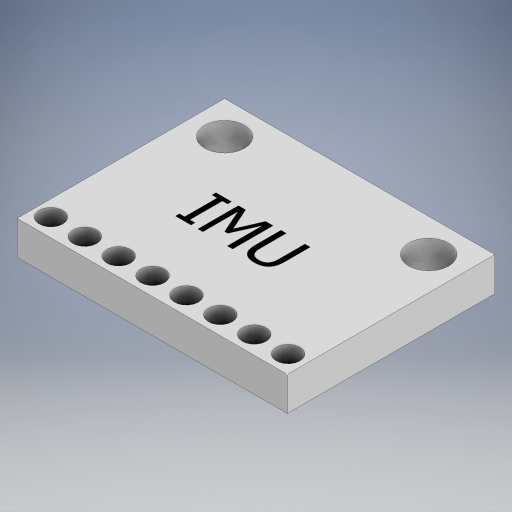
# Autodesk Inventor part: IMU_temp
Saved by Autodesk Inventor 2024 (Build 280153000, 153)
## iProperties
Created: 2025-01-15
Part Number: IMU_temp
Material: Generic
Document SubType Name: Modeling
Designer: Alex
Density: 1 g/cm^3
Appearance: Default
Author: Alex
Autodesk Inventor part; units mm, degrees
ref_plane "YZ Plane" through (0, 0, 0) normal (1, 0, 0) x (0, 1, 0)
ref_plane "XZ Plane" through (0, 0, 0) normal (0, 1, 0) x (-1, 0, 0)
ref_plane "XY Plane" through (0, 0, 0) normal (0, 0, 1) x (1, 0, 0)
sketch "Sketch1" plane through (0, 0, 0) normal (0, 1, 0) x (-1, 0, 0)
  line L0 (0, 0) -> (20.2618, 0)
  line L1 (20.2618, 0) -> (20.2618, -15.5601)
  line L2 (20.2618, -15.5601) -> (0, -15.5601)
  line L3 (0, -15.5601) -> (0, 0)
  dimension "d0" = 20.2618
  dimension "d1" = 15.5601
  constraints: 8 end point, 2 parallel, 1 horizontal, 1 perpendicular
  measures "d0" distance of L1.end L2.end
  measures "d1" distance of L0.end L1.end
extrude "Extrusion1" add sketch "Sketch1" along normal blind 2.54
sketch "Sketch2" plane through (0, 2.54, 0) normal (0, 1, 0) x (1, 0, 0)
  circle A0 centre (-19.0703, 1.3447) radius 0.8937
  line L0 (-20.2618, 15.5601) -> (-20.2618, 0) construction
  line L1 (-20.2618, 0) -> (0, 0) construction
  line L2 (-20.2618, 0) -> (0, 0) construction
  circle A1 centre (-16.5303, 1.3447) radius 0.8937
  circle A2 centre (-13.9903, 1.3447) radius 0.8937
  circle A3 centre (-11.4503, 1.3447) radius 0.8937
  circle A4 centre (-8.9103, 1.3447) radius 0.8937
  circle A5 centre (-6.3703, 1.3447) radius 0.8937
  circle A6 centre (-3.8303, 1.3447) radius 0.8937
  circle A7 centre (-1.2903, 1.3447) radius 0.8937
  circle A8 centre (-17.7809, 13.0792) radius 1.5
  circle A9 centre (-2.4809, 13.0792) radius 1.5
  line L3 (0, 15.5601) -> (-20.2618, 15.5601) projected
  line L4 (0, 0) -> (0, 15.5601) projected
  line L5 (-17.7809, 13.0792) -> (-2.4809, 13.0792) construction
  line L6 (-10.1309, 0) -> (-10.1309, 15.5601) construction
  point P0 (-10.1309, 13.0792)
  dimension "d6" = 2.54
  dimension "d11" = 3
  dimension "d12" = 3
  dimension "d17" = 15.3
  dimension "d18" = 2.4809
  dimension "d19" = 2.4809
  constraints: 10 centre point, 6 end point, 3 midpoint, 1 collinear, 1 horizontal, 1 perpendicular, 1 point on line, 14 other
  measures "d6" distance of A0.centre A1.centre
  measures "d11" diameter of A8
  measures "d12" diameter of A9
  measures "d17" distance of L5.end L5.start
  measures "d18" distance from line of L0 L5.start
  measures "d19" distance from line of L3 L5.start
extrude "Extrusion2" cut sketch "Sketch2" against normal up to next
sketch "Sketch3" plane through (0, 2.54, 0) normal (0, 1, 0) x (1, 0, 0)
  line L0 (-14.6694, 9.1277) -> (-2.5672, 9.1277) construction
  line L1 (-2.5672, 9.1277) -> (-2.5672, 4.9306) construction
  line L2 (-2.5672, 4.9306) -> (-14.6694, 4.9306) construction
  line L3 (-14.6694, 4.9306) -> (-14.6694, 9.1277) construction
  point P0 (0, 0)
  constraints: 2 other
equation "\"d19\" = d18"
body "Solid1"
